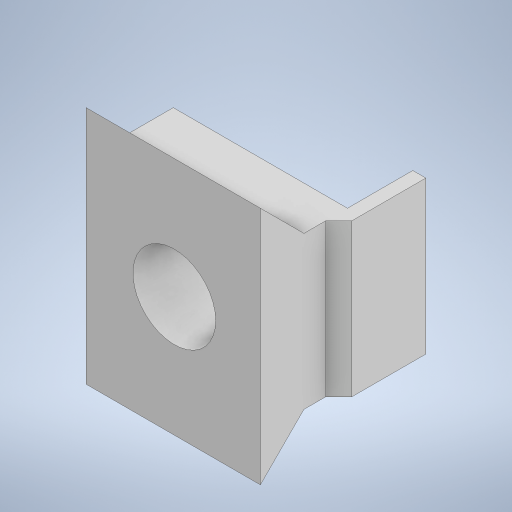
# Autodesk Inventor part: cam_mount
Saved by Autodesk Inventor 2024 (Build 280153000, 153)
## iProperties
Created: 2024-03-25
Part Number: cam_mount
Material: Generisch
Document SubType Name: Modeling
Designer: anash
Density: 1 g/cm^3
Appearance: Vorgabe
Author: anash
Autodesk Inventor part; units mm, degrees
ref_plane "YZ Plane" through (0, 0, 0) normal (1, 0, 0) x (0, 1, 0)
ref_plane "XZ Plane" through (0, 0, 0) normal (0, 1, 0) x (-1, 0, 0)
ref_plane "XY Plane" through (0, 0, 0) normal (0, 0, 1) x (1, 0, 0)
sketch "Skizze16" plane through (0, 0, 0) normal (0, 1, 0) x (-1, 0, 0)
  line L0 (0, 0) -> (-40, 0)
  line L1 (-40, 0) -> (-40, -65)
  line L2 (-40, -65) -> (0, -65)
  line L3 (0, -65) -> (0, 0)
  circle A0 centre (-20.25, -32.5) radius 3.25
  line L4 (-40, 0) -> (-43, 0)
  line L5 (-43, 0) -> (-43, -65)
  line L6 (-43, -65) -> (-40, -65)
  line L7 (-40, -65) -> (-40, 0)
  line L8 (0, 0) -> (-40, 0)
  line L9 (-40, 0) -> (-40, -15)
  line L10 (-40, -15) -> (0, -15)
  line L11 (0, -15) -> (0, 0)
  line L12 (0, -65) -> (-40, -65)
  line L13 (-40, -65) -> (-40, -50)
  line L14 (-40, -50) -> (0, -50)
  line L15 (0, -50) -> (0, -65)
  line L16 (-40, -15) -> (-43, -15)
  line L17 (-43, -15) -> (-43, -50)
  line L18 (-43, -50) -> (-40, -50)
  line L19 (-40, -50) -> (-40, -15)
  dimension "d88" = 40
  dimension "d89" = 65
  dimension "d90" = 19.75
  dimension "d91" = 32.5
  dimension "d92" = 6.5
  dimension "d93" = 3
  dimension "d113" = 15
  dimension "d114" = 15
  constraints: 40 end point, 10 parallel, 5 horizontal, 5 perpendicular, 3 point on line, 1 centre point
  measures "d88" distance of L2.end L1.end
  measures "d89" distance of L1.end L0.end
  measures "d90" distance from line of L1 A0.centre
  measures "d91" distance from line of L0 A0.centre
  measures "d92" diameter of A0
  measures "d93" distance of L6.end L5.end
  measures "d113" distance of L9.end L8.end
  measures "d114" distance of L12.end L13.end
extrude "Extrusion11" add sketch "Skizze16" along normal blind 5
sketch "Skizze17" plane through (0, 5, 0) normal (0, 1, 0) x (1, 0, 0)
  line L0 (0, 0) -> (43, 0) projected
  line L1 (43, 65) -> (0, 65) projected
  line L2 (43, 0) -> (40, 0)
  line L3 (40, 0) -> (40, 65)
  line L4 (40, 65) -> (43, 65)
  line L5 (43, 65) -> (43, 0)
  dimension "d96" = 3
  constraints: 8 end point, 2 parallel, 1 horizontal, 1 perpendicular, 1 point on line
  measures "d96" distance of L3.end L4.end
extrude "Extrusion12" add sketch "Skizze17" along normal blind 15
sketch "Skizze18" plane through (0, 0, 0) normal (0, -1, 0) x (1, 0, 0)
  line L0 (0, 0) -> (43, 0) projected
  line L1 (43, -65) -> (0, -65) projected
  line L2 (0, 0) -> (40, 0)
  line L3 (40, 0) -> (40, -65)
  line L4 (40, -65) -> (0, -65)
  line L5 (0, -65) -> (0, 0)
  circle A0 centre (20.25, -32.5) radius 3.25 projected
  circle A1 centre (20.25, -32.5) radius 3.25
  point P0 (0, -65)
  dimension "d99" = 40
  constraints: 8 end point, 2 parallel, 1 centre point, 1 coincident, 1 horizontal, 1 perpendicular, 1 point on line
  measures "d99" distance of L3.end L4.end
extrude "Extrusion13" add sketch "Skizze18" along normal blind 15
sketch "Skizze20" plane through (40, 0, 0) normal (1, 0, 0) x (0, 0, -1)
  line L0 (65, -15) -> (0, -15) projected
  line L1 (0, 0) -> (65, 0) projected
  line L2 (15, -15) -> (50, -15)
  line L3 (50, -15) -> (50, 0)
  line L4 (50, 0) -> (15, 0)
  line L5 (15, 0) -> (15, -15)
  line L6 (0, 0) -> (0, -15) projected
  line L7 (5, -15) -> (15, -5)
  line L8 (5, -15) -> (19.1421, -15) construction
  line L9 (60, -15) -> (50, -5)
  line L10 (60, -15) -> (74.1421, -15) construction
  line L11 (65, 5) -> (65, -15) projected
  line L12 (50, 0) -> (65, 0)
  line L13 (65, 0) -> (65, -15)
  line L14 (65, -15) -> (50, -15)
  line L15 (50, -15) -> (50, 0)
  point P0 (0, -7.5)
  point P1 (15, 0)
  dimension "d102" = 35
  dimension "d103" = 15
  dimension "d104" = 45
  dimension "d105" = 5
  dimension "d106" = 135
  dimension "d107" = 5
  constraints: 24 end point, 6 point on line, 4 horizontal, 4 parallel, 2 equal length, 2 perpendicular, 1 midpoint
  measures "d102" distance of L4.end L3.end
  measures "d103" distance from line of point (0, -7.5) L5
  measures "d104" angle of L8 L7
  measures "d105" distance of L0.end L7.start
  measures "d106" angle of L10 L9
  measures "d107" distance of L0.start L9.start
extrude "Extrusion14" cut sketch "Skizze20" against normal through all contours L0 L9 L3 L1 L11 | L5 L7 L0 L6 L1
chamfer "Fasen5" distance 3 angle 45 1 edges at (43, 0, -32.5)
sketch "Skizze21" plane through (0, 0, 0) normal (0, 0, 1) x (1, 0, 0)
  line L0 (0, 0) -> (0, 5) projected
  line L1 (0, 5) -> (0, 0)
  line L2 (40, 0) -> (40, -5) projected
  line L3 (0, 0) -> (40, 0)
  line L4 (40, 0) -> (43, 3) projected
  line L5 (40, 0) -> (43, 3)
  line L6 (43, 3) -> (43, 20) projected
  line L7 (43, 3) -> (43, 20)
  line L8 (40, 5) -> (40, 20) projected
  line L9 (43, 20) -> (40, 20)
  line L10 (40, 20) -> (40, 5)
  line L11 (40, 5) -> (0, 5)
  constraints: 14 end point, 4 perpendicular, 3 collinear
extrude "Extrusion15" cut sketch "Skizze21" against normal blind 15
sketch "Skizze22" plane through (0, 0, -65) normal (0, 0, -1) x (-1, 0, 0)
  line L0 (-40, 20) -> (-43, 20) projected
  line L1 (-43, 20) -> (-40, 20)
  line L2 (-40, 5) -> (-40, 20) projected
  line L3 (-40, 20) -> (-40, 5)
  line L4 (-40, 5) -> (0, 5)
  line L5 (0, 5) -> (0, 0)
  line L6 (0, -5) -> (0, 5) projected
  line L7 (0, 0) -> (-40, 0)
  line L8 (-40, 0) -> (-43, 3) projected
  line L9 (-40, 0) -> (-43, 3)
  line L10 (-43, 3) -> (-43, 20)
  line L11 (-40, 5) -> (-40, 20) projected
  constraints: 14 end point, 3 collinear, 1 horizontal, 1 parallel, 1 perpendicular
extrude "Extrusion16" cut sketch "Skizze22" against normal blind 15
sketch "Skizze24" plane through (0, -15, 0) normal (0, -1, 0) x (1, 0, 0)
  circle A0 centre (20.25, -32.5) radius 3.25 projected
  circle A1 centre (20.25, -32.5) radius 3.25
  circle A2 centre (20.25, -32.5) radius 5.75
  point P0 (0, 0)
  dimension "d119" = 11.5
  constraints: 2 centre point, 2 coincident
  measures "d119" diameter of A2
extrude "Extrusion17" cut sketch "Skizze24" against normal blind 14
chamfer "Fasen6" distance 3.75 angle 75 1 edges at (14.5, -15, -32.5)
